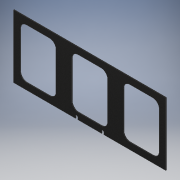
# Autodesk Inventor part: GBX_020.1-front-MDF
Saved by Autodesk Inventor 2019 (Build 230136000, 136)
## iProperties
Created: 2019-09-28
Part Number: GBX_020.1-front-MDF
Material: Generic
Document SubType Name: Modeling
Designer: Rene
Density: 1 g/cm^3
Appearance: Black Cast
Author: Rene
Autodesk Inventor part; units mm, degrees
ref_plane "YZ Plane" through (0, 0, 0) normal (1, 0, 0) x (0, 1, 0)
ref_plane "XZ Plane" through (0, 0, 0) normal (0, 1, 0) x (-1, 0, 0)
ref_plane "XY Plane" through (0, 0, 0) normal (0, 0, 1) x (1, 0, 0)
sketch "Sketch1" plane through (0, 0, 0) normal (0, 0, 1) x (1, 0, 0)
  line L0 (350, -145) -> (-350, -145)
  line L1 (-350, -145) -> (-350, 145)
  line L2 (-350, 145) -> (350, 145)
  line L3 (350, 145) -> (350, -145)
  line L4 (350, -145) -> (-350, 145) construction
  line L5 (-350, -145) -> (350, 145) construction
  point P0 (0, 0)
  dimension "d0" = 290
  dimension "d1" = 700
  constraints: 12 end point, 2 midpoint, 2 parallel, 1 horizontal, 1 perpendicular
  measures "d0" distance of L0.end L1.end
  measures "d1" distance of L1.end L2.end
extrude "Extrusion1" add sketch "Sketch1" along normal blind 3
sketch "Sketch2" plane through (0, 0, 3) normal (0, 0, 1) x (1, 0, 0)
  line L0 (-320, 115) -> (-155, 115)
  line L1 (-155, 115) -> (-155, -115)
  line L2 (-155, -115) -> (-320, -115)
  line L3 (-320, -115) -> (-320, 115)
  line L4 (-350, 145) -> (-350, -145) projected
  line L5 (350, 145) -> (-350, 145) projected
  line L6 (-350, -145) -> (350, -145) projected
  point P0 (0, 0)
  dimension "d4" = 30
  dimension "d5" = 30
  dimension "d6" = 30
  dimension "d7" = 165
  constraints: 8 end point, 2 parallel, 1 horizontal, 1 perpendicular
  measures "d4" distance between parallel lines of L3 L4
  measures "d5" distance between parallel lines of L5 L0
  measures "d6" distance between parallel lines of L2 L6
  measures "d7" distance of L0.start L0.end
extrude "Extrusion2" cut sketch "Sketch2" against normal blind 3
fillet "Fillet1" radius 30 4 edges at (-320, 115, 1.5) (-155, 115, 1.5) (-320, -115, 1.5) (-155, -115, 1.5)
mirror "Mirror1" about plane through (0, 0, 0) normal (1, 0, 0) of "Extrusion2", "Fillet1"
sketch "Sketch3" plane through (0, 0, 3) normal (0, 0, 1) x (1, 0, 0)
  line L0 (-290, 115) -> (-185, 115) projected
  line L1 (-155, 85) -> (-155, -85) projected
  line L2 (-185, -115) -> (-290, -115) projected
  line L3 (350, 145) -> (-350, 145) projected
  line L4 (-350, -145) -> (350, -145) projected
  line L5 (-350, 145) -> (-350, -145) projected
  line L6 (350, -145) -> (350, 145) projected
  line L7 (82.5, -115) -> (-82.5, -115)
  line L8 (-82.5, -115) -> (-82.5, 115)
  line L9 (-82.5, 115) -> (82.5, 115)
  line L10 (82.5, 115) -> (82.5, -115)
  line L11 (82.5, -115) -> (-82.5, 115) construction
  line L12 (-82.5, -115) -> (82.5, 115) construction
  line L13 (-320, -85) -> (-320, 85) projected
  point P0 (0, 0)
  dimension "d11" = 165
  dimension "d12" = 165
  constraints: 12 end point, 2 midpoint, 2 parallel, 1 horizontal, 1 perpendicular, 1 point on line
  measures "d11" distance between parallel lines of L1 L13
  measures "d12" distance between parallel lines of L10 L8
extrude "Extrusion3" cut sketch "Sketch3" against normal blind 3 contours L7 L8 L9 L10
fillet "Fillet2" radius 30 4 edges at (82.5, 115, 1.5) (-82.5, 115, 1.5) (-82.5, -115, 1.5) (82.5, -115, 1.5)
sketch "Sketch4" plane through (0, 0, 3) normal (0, 0, 1) x (1, 0, 0)
  line L0 (-350, 145) -> (-350, -145) projected
  line L1 (-350, -145) -> (350, -145) projected
  line L2 (-65, -145) -> (-55, -145)
  line L3 (-55, -145) -> (-55, -129.9972)
  line L4 (-55, -129.9972) -> (-65, -129.9972)
  line L5 (-65, -129.9972) -> (-65, -145)
  point P0 (0, 0)
  dimension "d16" = 285
  dimension "d17" = 10
  constraints: 8 end point, 2 parallel, 1 horizontal, 1 perpendicular, 1 point on line
  measures "d16" distance between parallel lines of L5 L0
  measures "d17" distance of L3.end L4.end
extrude "Extrusion4" cut sketch "Sketch4" against normal blind 3
fillet "Fillet3" radius 5 2 edges at (-65, -129.9972, 1.5) (-55, -129.9972, 1.5)
mirror "Mirror2" about plane through (0, 0, 0) normal (1, 0, 0) of "Extrusion4", "Fillet3"
equation "\"d12\" = d11"
equation "\"d20\" = 0.5 * d17"
body "Solid1"
